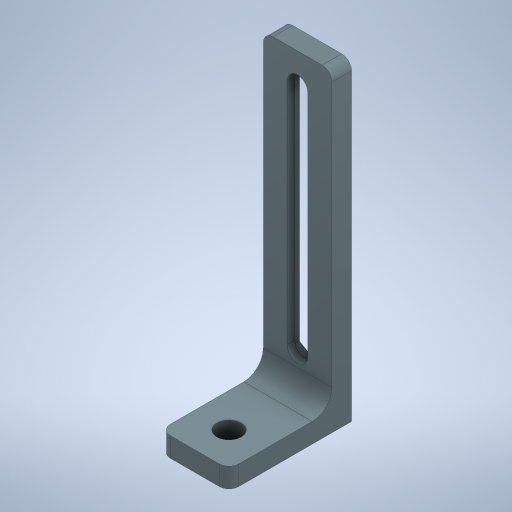
# Autodesk Inventor part: Sloupek
Saved by Autodesk Inventor 2024.2 (Build 282272000, 272)
## iProperties
Created: 2025-06-03
Part Number: Sloupek
Material: Olovo
Document SubType Name: Modeling
Designer: Elite
Density: 11.34 g/cm^3
Appearance: Olovo
Mass: 39.1257 g
Surface Area: 31.986 cm^2
Volume: 3.45024 cm^3
Author: Elite
Autodesk Inventor part; units mm, degrees
ref_plane "YZ Plane" through (0, 0, 0) normal (1, 0, 0) x (0, 1, 0)
ref_plane "XZ Plane" through (0, 0, 0) normal (0, 1, 0) x (-1, 0, 0)
ref_plane "XY Plane" through (0, 0, 0) normal (0, 0, 1) x (1, 0, 0)
sketch "Náčrt1" plane through (0, 0, 0) normal (0, 0, 1) x (1, 0, 0)
  line L0 (0, 0) -> (14, 0)
  line L1 (14, 0) -> (14, 25)
  line L2 (14, 25) -> (0, 25)
  line L3 (0, 25) -> (0, 0)
  circle A0 centre (7, 7) radius 2.5
  line L4 (0, 25) -> (14, 25)
  line L5 (14, 25) -> (14, 21)
  line L6 (14, 21) -> (0, 21)
  line L7 (0, 21) -> (0, 25)
  point P0 (0, 0)
  point P1 (7, 0)
  point P2 (0, 21)
  dimension "d0" = 14
  dimension "d1" = 25
  dimension "d2" = 5
  dimension "d3" = 7
  dimension "d4" = 7
  dimension "d5" = 4
  constraints: 16 end point, 4 parallel, 2 horizontal, 2 perpendicular, 1 centre point, 1 midpoint, 1 point on line
  measures "d0" distance of L2.end L1.end
  measures "d1" distance of L1.end L0.end
  measures "d2" diameter of A0
  measures "d3" distance from line of L3 A0.centre
  measures "d4" distance of point (7, 0) A0.centre
  measures "d5" distance between parallel lines of L6 L2
extrude "Vysunutí1" add sketch "Náčrt1" against normal blind 4
extrude "Vysunutí2" add sketch "Náčrt1" along normal blind 60 contours L3 L2 L1 L6
sketch "Náčrt2" plane through (0, 25, -4) normal (0, 1, 0) x (1, 0, 0)
  point P0 (0, -4)
sketch "Náčrt3" plane through (0, 25, -4) normal (0, 1, 0) x (1, 0, 0)
  line L0 (14, 0) -> (14, -64) projected
  line L1 (0, 0) -> (14, 0) projected
  line L2 (0, 0) -> (0, -64) projected
  line L3 (14, -64) -> (0, -64) projected
  line L4 (7, -6.7883) -> (10.6, -8.8668)
  line L5 (9.075, -57.6142) -> (9.075, -11.0396)
  line L6 (10.6, -59.7938) -> (7, -61.8722)
  line L7 (7, -61.8722) -> (3.4, -59.7938)
  line L8 (7, -61.8722) -> (3.4, -59.7938)
  line L9 (10.6, -59.7938) -> (7, -61.8722)
  line L10 (7, -6.7883) -> (10.6, -8.8668)
  arc A0 (4.925, -57.693) -> (9.075, -57.6142) centre (7.0012, -57.7147) ccw
  arc A1 (4.925, -57.693) -> (9.075, -57.6142) centre (7.0012, -57.7147) ccw
  line L11 (4.925, -11.0876) -> (4.925, -57.693)
  line L12 (9.075, -57.6142) -> (9.075, -11.0396)
  line L13 (10.6, -8.8668) -> (10.6, -59.7938)
  line L14 (10.6, -8.8668) -> (10.6, -59.7938)
  line L15 (3.4, -59.7938) -> (3.4, -8.8668)
  line L16 (3.4, -59.7938) -> (3.4, -8.8668)
  arc A2 (9.075, -11.0396) -> (4.925, -11.0876) centre (6.9987, -10.9484) ccw
  arc A3 (9.075, -11.0396) -> (4.925, -11.0876) centre (6.9987, -10.9484) ccw
  line L17 (3.4, -8.8668) -> (7, -6.7883)
  line L18 (3.4, -8.8668) -> (7, -6.7883)
  line L19 (4.925, -11.0876) -> (4.925, -57.693)
  point P0 (0, -4)
  point P1 (7, -8.87)
  point P2 (7, -8.87)
  point P3 (7, -64)
  point P4 (7.0406, -59.7906)
  dimension "d10" = 4.15
  dimension "d11" = 2.1278
  dimension "d12" = 2.0816
  dimension "d13" = 1.525
  constraints: 32 end point, 9 point on circle, 4 centre point, 1 midpoint
  measures "d10" distance between parallel lines of L5 L11
  measures "d11" distance of point (7, -64) L9.end
  measures "d12" vertical distance of L9.end point (7.041, -59.791)
  measures "d13" distance between parallel lines of L19 L16
extrude "Vysunutí3" cut sketch "Náčrt3" against normal blind 60 contours A0 L11 A2 L5
extrude "Vysunutí4" cut sketch "Náčrt3" against normal blind 2.5 contours L4 L13 L6 L7 L15 L17
fillet "Zaoblení1" radius 2 2 edges at (14, 23, 60) (0, 23, 60)
fillet "Zaoblení2" radius 2 2 edges at (14, 0, -2) (0, 0, -2)
fillet "Zaoblení3" radius 4 1 edges at (7, 21, 0)
